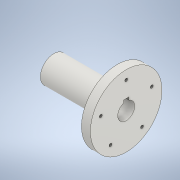
# Autodesk Inventor part: Sprocket_Rueda
Saved by Autodesk Inventor 2022.1 (Build 261234000, 234)
## iProperties
Created: 2021-09-22
Part Number: Sprocket_Rueda
Material: Genérico
Document SubType Name: Modeling
Designer: seb_0
Density: 1 g/cm^3
Appearance: Acero
Author: seb_0
Autodesk Inventor part; units mm, degrees
ref_plane "YZ Plane" through (0, 0, 0) normal (1, 0, 0) x (0, 1, 0)
ref_plane "XZ Plane" through (0, 0, 0) normal (0, 1, 0) x (-1, 0, 0)
ref_plane "XY Plane" through (0, 0, 0) normal (0, 0, 1) x (1, 0, 0)
sketch "Boceto1" plane through (0, 0, 0) normal (1, 0, 0) x (0, 1, 0)
  circle A0 centre (0, 0) radius 40
  circle A1 centre (0, 0) radius 30
  circle A2 centre (30, 0) radius 1.25
  circle A3 centre (9.2705, 28.5317) radius 1.25
  circle A4 centre (-24.2705, -17.6336) radius 1.25
  circle A5 centre (-24.2705, 17.6336) radius 1.25
  line L0 (0, 0) -> (30, 0)
  line L1 (0, 0) -> (9.2705, -28.5317)
  line L2 (0, 0) -> (-24.2705, -17.6336)
  line L3 (0, 0) -> (-24.2705, 17.6336)
  line L4 (0, 0) -> (9.2705, 28.5317)
  circle A6 centre (9.2705, -28.5317) radius 1.25
  dimension "d0" = 80
  dimension "d1" = 60
  dimension "d7" = 72
  dimension "d8" = 72
  dimension "d9" = 72
  dimension "d10" = 72
  dimension "d24" = 2.5
  constraints: 10 end point, 7 centre point, 5 point on circle, 4 equal radius, 3 coincident, 1 horizontal
  measures "d0" diameter of A0
  measures "d1" diameter of A1
  measures "d7" angle of L1 L0
  measures "d8" angle of L2 L1
  measures "d9" angle of L3 L2
  measures "d10" angle of L4 L3
  measures "d24" diameter of A2
extrude "Extrusión1" add sketch "Boceto1" along normal blind 10 contours A0 | A2 L0 L4 A3 A1 | A1 A6 L1 L0 A2 | L1 A6 A1 A4 L2 | L2 A4 A1 A5 L3 | L3 A5 A1 A3 L4
sketch "Boceto2" plane through (0, 0, 0) normal (-1, 0, 0) x (0, 0, 1)
  circle A0 centre (0, 0) radius 15
  dimension "d14" = 30
  constraints: 1 centre point, 1 coincident
  measures "d14" diameter of A0
extrude "Extrusión2" add sketch "Boceto2" along normal blind 71
sketch "Boceto3" plane through (-71, 0, 0) normal (-1, 0, 0) x (0, 0, 1)
  circle A0 centre (0, 0) radius 9.5
  line L0 (-3, 12) -> (3, 12)
  line L1 (3, 12) -> (3, 0)
  line L2 (3, 0) -> (-3, 0)
  line L3 (-3, 0) -> (-3, 12)
  point P0 (-3, 9.0139)
  point P1 (3, 9.0139)
  dimension "d17" = 19
  dimension "d18" = 6
  dimension "d19" = 12
  dimension "d20" = 12
  dimension "d21" = 3
  constraints: 8 end point, 2 parallel, 1 centre point, 1 coincident, 1 horizontal, 1 perpendicular
  measures "d17" diameter of A0
  measures "d18" distance of L0.start L0.end
  measures "d19" distance of L0.end L1.end
  measures "d20" distance from line of point (0, 0) L0
  measures "d21" distance from line of point (0, 0) L3
extrude "Extrusión3" cut sketch "Boceto3" against normal through all
sketch "Boceto4" plane through (10, 0, 0) normal (1, 0, 0) x (0, 0, -1)
  arc A0 (-3, 9.0139) -> (3, 9.0139) centre (0, 0) ccw projected
  line L0 (-3, 9.0139) -> (-3, 12) projected
  line L1 (-3, 12) -> (3, 12) projected
  line L2 (3, 12) -> (3, 9.0139) projected
  circle A1 centre (0, 0) radius 40 projected
  circle A2 centre (0, 30) radius 1.25 projected
  circle A3 centre (-28.5317, 9.2705) radius 1.25 projected
  circle A4 centre (17.6336, -24.2705) radius 1.25 projected
  circle A5 centre (-17.6336, -24.2705) radius 1.25 projected
  circle A6 centre (28.5317, 9.2705) radius 1.25 projected
hole "Agujero1" at (10, 30, 0) at (10, 9.2705, -28.5317) at (10, -24.2705, -17.6336) at (10, 9.2705, 28.5317) at (10, -24.2705, 17.6336) direction (-1, 0, 0) diameter 3.242 end through all thread size "M4x0.7" class "6H" standard "ANSI Metric M Profile"
